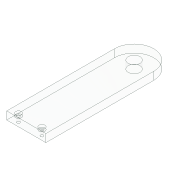
# Autodesk Inventor part: Bearing10
Saved by Autodesk Inventor 2022.5 (Build 265521000, 521)
## iProperties
Created: 2020-02-29
Part Number: Bearing10
Document SubType Name: Modeling
Designer: Administrator
Density: 1 g/cm^3
Material: Generic
Appearance: Clear
Author: Administrator
Autodesk Inventor part; units mm, degrees
ref_plane "YZ Plane" through (0, 0, 0) normal (1, 0, 0) x (0, 1, 0)
ref_plane "XZ Plane" through (0, 0, 0) normal (0, 1, 0) x (-1, 0, 0)
ref_plane "XY Plane" through (0, 0, 0) normal (0, 0, 1) x (1, 0, 0)
sketch "Sketch1" plane through (0, 0, 0) normal (0, 0, 1) x (1, 0, 0)
  circle A0 centre (0, 0) radius 6
  line L0 (20, 20) -> (20, -20)
  line L1 (20, -20) -> (-20, -20)
  line L2 (-20, -20) -> (-20, 20)
  line L3 (-20, 20) -> (20, 20)
  line L4 (-20, -20) -> (20, -20)
  line L5 (20, -20) -> (20, -110)
  line L6 (20, -110) -> (-20, -110)
  line L7 (-20, -110) -> (-20, -20)
  dimension "d0" = 12
  dimension "d1" = 40
  dimension "d5" = 110
  constraints: 16 end point, 3 parallel, 1 centre point, 1 coincident, 1 horizontal, 1 perpendicular, 1 vertical, 10 other
  measures "d0" diameter of A0
  measures "d1" distance of L2.end L0.start
  measures "d5" distance from line of A0.centre L6
extrude "Extrusion1" add sketch "Sketch1" along normal blind 8
fillet "Fillet1" radius 20 2 edges at (20, 20, 4) (-20, 20, 4)
sketch "Sketch2" plane through (0, 0, 8) normal (0, 0, 1) x (1, 0, 0)
  line L0 (20, -110) -> (-20, -110) construction
  line L1 (-20, -110) -> (-20, 0) construction
  line L2 (20, 0) -> (20, -110) construction
  line L3 (-20, -110) -> (20, -110) construction
  line L4 (20, -110) -> (20, -102) construction
  line L5 (20, -102) -> (-20, -102) construction
  line L6 (-20, -102) -> (-20, -110) construction
  line L7 (0, -102) -> (0, -110) construction
  line L8 (0, -106) -> (-12, -106) construction
  circle A0 centre (-12, -106) radius 1.5
  point P0 (0, 0)
  dimension "d7" = 8
  dimension "d8" = 3
  dimension "d14" = 12
  constraints: 12 end point, 3 midpoint, 2 horizontal, 2 parallel, 1 centre point, 1 coincident, 1 perpendicular, 1 point on line
  measures "d7" distance between parallel lines of L0 L5
  measures "d8" diameter of A0
  measures "d14" distance of L8.start L8.end
extrude "Extrusion2" cut sketch "Sketch2" against normal through all
sketch "Sketch3" plane through (0, 0, 8) normal (0, 0, 1) x (1, 0, 0)
  circle A0 centre (-12, -106) radius 1.5 projected
  circle A1 centre (-12, -106) radius 3
  point P0 (0, 0)
  dimension "d11" = 6
  constraints: 1 centre point
  measures "d11" diameter of A1
extrude "Extrusion3" cut sketch "Sketch3" against normal blind 2.5
mirror "Mirror1" about plane through (0, 0, 0) normal (1, 0, 0) of "Extrusion2", "Extrusion3"
body "Solid1"
